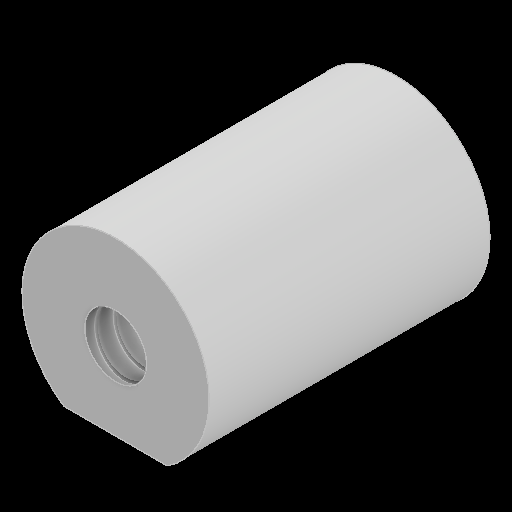
# Autodesk Inventor part: ShaftD6Female-632Female
Saved by Autodesk Inventor 2025.2 (Build 292293000, 293)
## iProperties
Created: 2021-07-06
Part Number: ShaftD6Female-632Female
Material: Generic
Document SubType Name: Modeling
Designer: Val
Density: 1 g/cm^3
Appearance: Default
Author: Val
Autodesk Inventor part; units mm, degrees
ref_plane "YZ Plane" through (0, 0, 0) normal (1, 0, 0) x (0, 1, 0)
ref_plane "XZ Plane" through (0, 0, 0) normal (0, 1, 0) x (-1, 0, 0)
ref_plane "XY Plane" through (0, 0, 0) normal (0, 0, 1) x (1, 0, 0)
sketch "Base" plane through (0, 0, 0) normal (0, 0, 1) x (1, 0, 0)
  line L0 (-1.6583, -2.2561) -> (1.6583, -2.2561)
  arc A0 (1.6583, -2.2561) -> (-1.6583, -2.2561) centre (0, 0) ccw
  arc A1 (2.2111, -3.3333) -> (-2.2111, -3.3333) centre (0, 0) ccw
  line L1 (2.2111, -3.3333) -> (-2.2111, -3.3333)
  line L2 (-5.6, 0) -> (5.6, 0) construction
  dimension "d1" = 2.8
  dimension "d2" = 3.3166
  dimension "d22" = 4
  dimension "d23" = 3.3333
  constraints: 4 end point, 4 point on circle, 2 centre point, 1 coincident, 1 horizontal, 1 parallel
  measures "d1" radius of A0
  measures "d2" distance of L0.start L0.end
  measures "d22" radius of A1
  measures "d23" distance between parallel lines of L1 L2
extrude "BaseFeature" add sketch "Base" along normal blind 12
sketch "Mount" plane through (0, 0, 12) normal (0, 0, 1) x (1, 0, 0)
  arc A0 (2.2111, -3.3333) -> (-2.2111, -3.3333) centre (0, 0) ccw projected
  line L0 (-2.2111, -3.3333) -> (2.2111, -3.3333) projected
extrude "MountFeature" add sketch "Mount" against normal blind 6.35
sketch "MountHole" plane through (0, 0, 12) normal (0, 0, 1) x (1, 0, 0)
  point P0 (0, 0)
hole "MountHoleFeature" at (0, 0, 12) direction (0, 0, -1) diameter 2.6416 end through all thread size "6-32 UNC" class "2B" standard "ANSI Unified Screw Threads"
body "Solid1"
